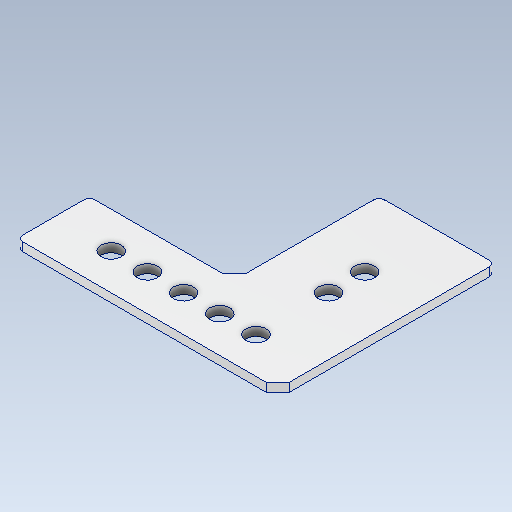
# Autodesk Inventor part: TopGussetPlate
Saved by Autodesk Inventor 2020 (Build 240168000, 168)
## iProperties
Created: 2021-01-20
Part Number: TopGussetPlate
Material: Aluminum 6061
Document SubType Name: Modeling
Designer: lucky
Density: 2.7 g/cm^3
Appearance: Aluminum - Flat
Mass: 32.2151 g
Surface Area: 93.818 cm^2
Volume: 11.9315 cm^3
Author: lucky
Autodesk Inventor part; units mm, degrees
ref_plane "YZ Plane" through (0, 0, 0) normal (1, 0, 0) x (0, 1, 0)
ref_plane "XZ Plane" through (0, 0, 0) normal (0, 1, 0) x (-1, 0, 0)
ref_plane "XY Plane" through (0, 0, 0) normal (0, 0, 1) x (1, 0, 0)
sketch "Sketch1" plane through (0, 0, 0) normal (0, 1, 0) x (-1, 0, 0)
  line L0 (-16, 12.5) -> (68, 12.5)
  line L1 (70, 10.5) -> (70, -10.5)
  line L2 (68, -12.5) -> (24, -12.5)
  line L3 (-20, -12.5) -> (-20, 8.5)
  line L4 (-20, -12.5) -> (20, -12.5)
  line L5 (20, -16.5) -> (20, -60.5)
  line L6 (18, -62.5) -> (-18, -62.5)
  line L7 (-20, -60.5) -> (-20, -12.5)
  line L8 (20, -16.5) -> (24, -12.5)
  line L9 (-20, 8.5) -> (-16, 12.5)
  arc A0 (-20, -60.5) -> (-18, -62.5) centre (-18, -60.5) ccw
  arc A1 (18, -62.5) -> (20, -60.5) centre (18, -60.5) ccw
  arc A2 (70, 10.5) -> (68, 12.5) centre (68, 10.5) ccw
  arc A3 (68, -12.5) -> (70, -10.5) centre (68, -10.5) ccw
  point P0 (0, 0)
  point P1 (-20, 12.5)
  point P2 (70, -12.5)
  point P3 (70, 12.5)
  point P4 (20, -62.5)
  point P5 (-20, -62.5)
  point P6 (0, -62.5)
  point P7 (70, 0)
  point P8 (20, -12.5)
  dimension "d0" = 40
  dimension "d1" = 25
  dimension "d2" = 50
  dimension "d3" = 50
  dimension "d22" = 4
  dimension "d23" = 4
  dimension "d24" = 4
  dimension "d25" = 4
  dimension "d26" = 2
  constraints: 20 end point, 14 point on line, 8 point on circle, 8 tangent, 4 centre point, 4 parallel, 3 equal radius, 2 horizontal, 2 midpoint, 2 perpendicular, 1 horizontal alignment, 1 vertical alignment
  measures "d0" distance between parallel lines of L7 L5
  measures "d1" distance between parallel lines of L2 L0
  measures "d2" distance between parallel lines of L5 L1
  measures "d3" distance from line of point (0, -62.5) L2
  measures "d22" distance of L5.start point (20, -12.5)
  measures "d23" distance of L2.end point (20, -12.5)
  measures "d24" distance of L3.end point (-20, 12.5)
  measures "d25" distance of L0.start point (-20, 12.5)
  measures "d26" radius of A0
extrude "Extrusion1" add sketch "Sketch1" along normal blind 3
sketch "Sketch2" plane through (0, 3, 0) normal (0, 1, 0) x (1, 0, 0)
  line L0 (20, -8.5) -> (20, 60.5) projected
  line L1 (18, 62.5) -> (-18, 62.5) projected
  line L2 (-20, 60.5) -> (-20, 16.5) projected
  line L3 (-24, 12.5) -> (-68, 12.5) projected
  line L4 (-70, 10.5) -> (-70, -10.5) projected
  line L5 (-68, -12.5) -> (16, -12.5) projected
  line L6 (20, 62.5) -> (-20, 62.5) projected
  line L7 (-20, 16.5) -> (-24, 12.5) projected
  arc A0 (-68, 12.5) -> (-70, 10.5) centre (-68, 10.5) ccw projected
  arc A1 (-70, -10.5) -> (-68, -12.5) centre (-68, -10.5) ccw projected
  line L8 (16, -12.5) -> (20, -8.5) projected
  arc A2 (20, 60.5) -> (18, 62.5) centre (18, 60.5) ccw projected
  arc A3 (-18, 62.5) -> (-20, 60.5) centre (-18, 60.5) ccw projected
  point P0 (0, 0)
  point P1 (0, 0)
  point P2 (0, 25)
  point P3 (0, 37.5)
  point P4 (-12.5, 0)
  point P5 (-25, 0)
  point P6 (-37.5, 0)
  point P7 (-50, 0)
  point P8 (0, 62.5)
  point P9 (0, 62.5)
  dimension "d8" = 12.5
  dimension "d13" = 25
  dimension "d14" = 12.5
  constraints: 2 midpoint, 2 vertical alignment, 1 coincident, 1 horizontal, 4 other
  measures "d8" distance of point (0, 0) point (-12.5, 0)
  measures "d13" distance of point (0, 25) point (0, 0)
  measures "d14" distance of point (0, 37.5) point (0, 25)
hole "Hole1" at (0, 3, 0) at (0, 3, -25) at (0, 3, -37.5) at (-50, 3, 0) at (-37.5, 3, 0) at (-25, 3, 0) at (-12.5, 3, 0) direction (0, -1, 0) diameter 7 depth 8
equation "\"d23\" = d22"
equation "\"d25\" = d24"
body "Solid1"
